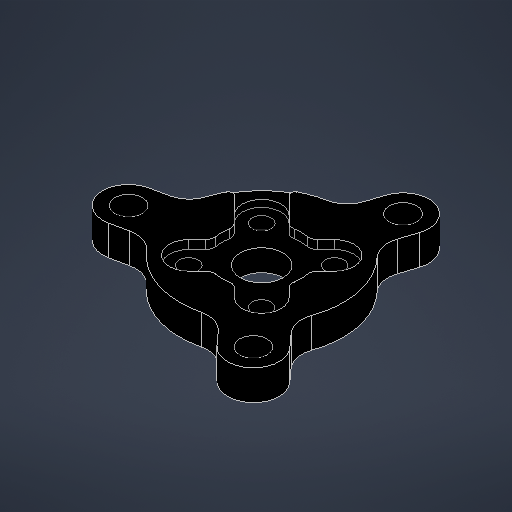
# Autodesk Inventor part: Motor Mounting Plate
Saved by Autodesk Inventor 2026.1 (Build 301233020, 233B)
## iProperties
Created: 2026-04-17
Part Number: Motor Mounting Plate
Material: Generic
Document SubType Name: Modeling
Designer: Bahaa
Mass: 1.06448 g
Surface Area: 12.4872 cm^2
Volume: 1.06448 cm^3
Density: 1 g/cm^3
Appearance: Black PLA
Author: Bahaa
Autodesk Inventor part; units mm, degrees
ref_plane "YZ Plane" through (0, 0, 0) normal (1, 0, 0) x (0, 1, 0)
ref_plane "XZ Plane" through (0, 0, 0) normal (0, 1, 0) x (-1, 0, 0)
ref_plane "XY Plane" through (0, 0, 0) normal (0, 0, 1) x (1, 0, 0)
sketch "Sketch1" plane through (0, 0, 0) normal (0, 0, 1) x (1, 0, 0)
  circle A0 centre (0, 0) radius 9.5
  circle A1 centre (0, 0) radius 4.625
  circle A2 centre (0, 6) radius 2.25
  line L0 (-2.25, 6) -> (-2.25, 4.0408)
  line L1 (2.25, 6) -> (2.25, 4.0408)
  circle A3 centre (0, 0) radius 2.5
  circle A4 centre (-4.2426, 4.2426) radius 2.25
  line L2 (-2.6517, 5.8336) -> (-1.2663, 4.4483)
  line L3 (-5.8336, 2.6517) -> (-4.4483, 1.2663)
  circle A5 centre (-6, 0) radius 2.25
  line L4 (-6, 2.25) -> (-4.0408, 2.25)
  line L5 (-6, -2.25) -> (-4.0408, -2.25)
  circle A6 centre (-4.2426, -4.2426) radius 2.25
  line L6 (-5.8336, -2.6517) -> (-4.4483, -1.2663)
  line L7 (-2.6517, -5.8336) -> (-1.2663, -4.4483)
  circle A7 centre (0, -6) radius 2.25
  line L8 (-2.25, -6) -> (-2.25, -4.0408)
  line L9 (2.25, -6) -> (2.25, -4.0408)
  circle A8 centre (4.2426, -4.2426) radius 2.25
  line L10 (2.6517, -5.8336) -> (1.2663, -4.4483)
  line L11 (5.8336, -2.6517) -> (4.4483, -1.2663)
  circle A9 centre (6, 0) radius 2.25
  line L12 (6, -2.25) -> (4.0408, -2.25)
  line L13 (6, 2.25) -> (4.0408, 2.25)
  circle A10 centre (4.2426, 4.2426) radius 2.25
  line L14 (5.8336, 2.6517) -> (4.4483, 1.2663)
  line L15 (2.6517, 5.8336) -> (1.2663, 4.4483)
  circle A11 centre (8.7322, -9.698) radius 3
  line L16 (0, 0) -> (8.7322, -9.698) construction
  line L17 (-9.5, 0) -> (9.5, 0) construction
  circle A12 centre (8.7322, -9.698) radius 1.6
  line L18 (6.5027, -11.7054) -> (3.802, -8.706)
  line L19 (10.9616, -7.6906) -> (8.2609, -4.6912)
  line L20 (6.8858, 11.4842) -> (5.6386, 7.6457)
  circle A13 centre (4.0327, 12.4113) radius 3
  circle A14 centre (4.0327, 12.4113) radius 1.6
  line L21 (1.1795, 13.3383) -> (-0.0677, 9.4998)
  line L22 (-13.3886, 0.2212) -> (-9.4406, 1.0604)
  circle A15 centre (-12.7648, -2.7132) radius 3
  circle A16 centre (-12.7648, -2.7132) radius 1.6
  line L23 (-12.1411, -5.6477) -> (-8.1932, -4.8085)
  line L24 (-5.8336, 2.6517) -> (-8.1174, 4.9354)
  line L25 (-2.6517, 5.8336) -> (-4.9354, 8.1174)
  point P0 (-4.4483, 1.2663)
  point P1 (-4.4483, -1.2663)
  point P2 (-1.2663, -4.4483)
  point P3 (1.2663, -4.4483)
  point P4 (4.4483, -1.2663)
  point P5 (4.4483, 1.2663)
  point P6 (1.2663, 4.4483)
  point P7 (-1.2663, 4.4483)
  point P8 (-12.1411, -5.6477)
  point P9 (-8.1932, -4.8085)
  point P10 (-9.4406, 1.0604)
  point P11 (10.9616, -7.6906)
  point P12 (8.2609, -4.6912)
  point P13 (1.1795, 13.3383)
  point P14 (-0.0677, 9.4998)
  point P15 (5.6386, 7.6457)
  dimension "d20" = 6
  dimension "d0" = 19
  dimension "d1" = 9.25
  dimension "d2" = 4.5
  dimension "d3" = 6
  dimension "d4" = 5
  dimension "d7" = 360
  dimension "d21" = 13.05
  dimension "d22" = 48
  dimension "d23" = 3.2
  dimension "d27" = 360
  constraints: 52 end point, 22 point on circle, 14 centre point, 6 coincident, 4 tangent, 3 parallel, 2 symmetric about line, 1 horizontal, 1 midpoint, 1 vertical, 1 vertical alignment, 106 other
  measures "d0" diameter of A0
  measures "d1" diameter of A1
  measures "d2" diameter of A2
  measures "d3" distance of point (0, 0) A2.centre
  measures "d4" diameter of A3
  measures "d21" distance of A0.centre L16.end
  measures "d22" angle of L17 L16
  measures "d23" diameter of A12
extrude "Extrusion1" add sketch "Sketch1" against normal blind 3.5
extrude "Extrusion2" cut sketch "Sketch1" against normal blind 1 contours A4 L0 A1 L4 | L2 L0 A4 | A4 L4 L3 | A4 A1 L0 | L0 L2 A2 A1 A4 | L4 A1 A4 | A4 A1 A5 L3 L4 | A1 A4 | L2 A1 A2 | A4 A1 A2 A10 A9 A8 A7 A6 A5 | A5 A1 L3 | A1 A2 | A5 A1 | L15 L1 A10 A1 A2 | A2 A1 L15 | L15 A10 L1 | A1 A5 L6 | A5 A1 A6 L5 L6 | L5 A6 L6 | A10 L13 A1 L1 | L1 A1 A10 | A1 A10 | A6 A1 L5 | L5 A1 L8 A6 | A10 L13 L14 A9 A1 | A1 L13 A10 | A6 A1 | A6 L8 L7 | L14 L13 A10 | A9 L14 A1 | A1 A9 | A6 L8 A1 | A1 A7 L7 L8 A6 | A9 L11 L12 A8 A1 | A1 L11 A9 | A7 A1 | A1 L7 A7 | A8 L12 A1 | A1 A8 | A7 L10 A1 | A1 A8 L9 L10 A7 | L12 A8 L9 A1 | L12 L11 A8 | A1 L9 A8 | L9 A8 L10 | A3
sketch "Sketch2" plane through (0, 0, -3.5) normal (0, 0, -1) x (-1, 0, 0)
  point P0 (-4.2426, -4.2426)
  point P1 (4.2426, -4.2426)
  point P2 (-4.2426, 4.2426)
  point P3 (4.2426, 4.2426)
hole "Hole1" at (4.2426, 4.2426, -3.5) at (-4.2426, 4.2426, -3.5) at (4.2426, -4.2426, -3.5) at (-4.2426, -4.2426, -3.5) direction (0, 0, 1) diameter 2.2 end through all countersink diameter 4.4 countersink angle 90 clearance for "Countersunk Flat Head Screw DIN EN ISO 2009" size "M2" standard "DIN"
fillet "Fillet1" radius 3 6 edges at (-8.1932, -4.8085, -1.75) (-9.4406, 1.0604, -1.75) (-0.0677, 9.4998, -1.75) (5.6386, 7.6457, -1.75) (8.2609, -4.6912, -1.75) (3.802, -8.706, -1.75)
fillet "Fillet2" radius 1 8 edges at (-4.4483, -1.2663, -0.5) (-4.4483, 1.2663, -0.5) (-1.2663, -4.4483, -0.5) (1.2663, -4.4483, -0.5) (-1.2663, 4.4483, -0.5) (1.2663, 4.4483, -0.5) (4.4483, 1.2663, -0.5) (4.4483, -1.2663, -0.5)
extrude "Extrusion3" cut sketch "Sketch1" against normal blind 0.2 contours L25 A4 L24 A0
fillet "Fillet3" radius 0.5 2 edges at (-8.1174, 4.9354, -0.1) (-4.9354, 8.1174, -0.1)
body "Solid1"
